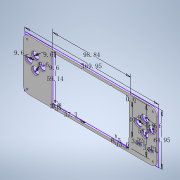
# Autodesk Inventor part: shell_panel
Saved by Autodesk Inventor 2022 (Build 260153000, 153)
## iProperties
Created: 2022-07-04
Part Number: shell_panel
Material: 常规
Document SubType Name: Modeling
Designer: yangmc
Density: 1 g/cm^3
Appearance: 默认
Author: yangmc
Autodesk Inventor part; units mm, degrees
ref_plane "YZ Plane" through (0, 0, 0) normal (1, 0, 0) x (0, 1, 0)
ref_plane "XZ Plane" through (0, 0, 0) normal (0, 1, 0) x (-1, 0, 0)
ref_plane "XY Plane" through (0, 0, 0) normal (0, 0, 1) x (1, 0, 0)
sketch "草图1" plane through (0, 0, 0) normal (0, 0, 1) x (1, 0, 0)
  circle A0 centre (15.38, 47) radius 4.8
  circle A1 centre (7.13, 38.85) radius 4.8
  circle A2 centre (15.38, 30.6) radius 4.8
  circle A3 centre (23.63, 38.85) radius 4.8
  circle A4 centre (154.65, 47) radius 4.8
  circle A5 centre (154.65, 30.5) radius 4.8
  circle A6 centre (162.9, 38.75) radius 4.8
  circle A7 centre (146.4, 38.75) radius 4.8
  line L0 (160.06, 15.83) -> (164.06, 15.83) construction
  line L1 (145.2, 15.83) -> (149.2, 15.83) construction
  line L2 (35.58, 3.33) -> (134.42, 3.33)
  line L3 (134.42, 3.33) -> (134.42, 61.67)
  line L4 (134.42, 61.67) -> (35.58, 61.67)
  line L5 (35.58, 61.67) -> (35.58, 3.33)
  line L6 (37.0724, 3.33) -> (39.6724, 3.33)
  line L7 (39.6724, 3.33) -> (39.6724, 2.53)
  line L8 (39.6724, 2.53) -> (37.0724, 2.53)
  line L9 (37.0724, 2.53) -> (37.0724, 3.33)
  line L10 (76.9724, 2.53) -> (74.3724, 2.53)
  line L11 (74.3724, 3.33) -> (76.9724, 3.33)
  line L12 (76.9724, 3.33) -> (76.9724, 2.53)
  line L13 (74.3724, 2.53) -> (74.3724, 3.33)
  line L14 (114.2724, 2.53) -> (111.6724, 2.53)
  line L15 (111.6724, 3.33) -> (114.2724, 3.33)
  line L16 (114.2724, 3.33) -> (114.2724, 2.53)
  line L17 (111.6724, 2.53) -> (111.6724, 3.33)
  line L18 (39.6724, 61.67) -> (37.0724, 61.67)
  line L19 (37.0724, 62.47) -> (39.6724, 62.47)
  line L20 (39.6724, 62.47) -> (39.6724, 61.67)
  line L21 (37.0724, 61.67) -> (37.0724, 62.47)
  line L22 (76.9724, 61.67) -> (74.3724, 61.67)
  line L23 (74.3724, 62.47) -> (76.9724, 62.47)
  line L24 (76.9724, 62.47) -> (76.9724, 61.67)
  line L25 (74.3724, 61.67) -> (74.3724, 62.47)
  line L26 (114.2724, 61.67) -> (111.6724, 61.67)
  line L27 (111.6724, 62.47) -> (114.2724, 62.47)
  line L28 (114.2724, 62.47) -> (114.2724, 61.67)
  line L29 (111.6724, 61.67) -> (111.6724, 62.47)
  line L30 (131.74, 3.33) -> (116.14, 3.33)
  line L31 (116.14, 3.33) -> (116.14, 2.83)
  line L32 (116.14, 2.83) -> (131.74, 2.83)
  line L33 (131.74, 2.83) -> (131.74, 3.33)
  line L34 (134.42, 16.2898) -> (135.02, 16.2898)
  line L35 (134.42, 43.8944) -> (134.42, 16.2898)
  line L36 (0.05, 0.05) -> (170, 0.05)
  line L37 (170, 0.05) -> (170, 65)
  line L38 (170, 65) -> (0.05, 65)
  line L39 (0.05, 65) -> (0.05, 0.05)
  line L40 (51, 0.05) -> (56.35, 0.05)
  line L41 (74.3724, 61.67) -> (76.72, 61.67)
  line L42 (143.65, 15.83) -> (150.75, 15.83) construction
  line L43 (145.2, 14.28) -> (149.2, 14.28)
  line L44 (149.2, 17.38) -> (145.2, 17.38)
  arc A8 (145.2, 17.38) -> (145.2, 14.28) centre (145.2, 15.83) ccw
  arc A9 (149.2, 14.28) -> (149.2, 17.38) centre (149.2, 15.83) ccw
  line L45 (158.51, 15.83) -> (165.61, 15.83) construction
  line L46 (160.06, 14.28) -> (164.06, 14.28)
  line L47 (164.06, 17.38) -> (160.06, 17.38)
  arc A10 (160.06, 17.38) -> (160.06, 14.28) centre (160.06, 15.83) ccw
  arc A11 (164.06, 14.28) -> (164.06, 17.38) centre (164.06, 15.83) ccw
  line L48 (135.02, 16.2898) -> (135.02, 56.2898)
  line L49 (135.02, 56.2898) -> (134.42, 56.2898)
  point P0 (0, 0)
  point P1 (162.06, 15.83)
  point P2 (147.2, 15.83)
  point P3 (72.9763, 65)
  point P4 (51, 0)
  point P5 (56.35, 0)
  point P6 (87, 65)
  point P7 (73, 65)
  point P8 (0, 0)
  point P9 (1.44, 58.34)
  point P10 (3.94, 58.34)
  point P11 (38.84, 58.34)
  point P12 (41.34, 58.34)
  point P13 (76.24, 58.34)
  point P14 (78.74, 58.34)
  point P15 (78.74, 0)
  point P16 (76.24, 0)
  point P17 (41.34, 0)
  point P18 (38.84, 0)
  point P19 (3.94, 0)
  point P20 (1.44, 0)
  point P21 (96.16, 0)
  point P22 (80.56, 0)
  point P23 (98.84, 43.1523)
  point P24 (37.02, 61.67)
  point P25 (39.52, 61.67)
  point P26 (74.42, 61.67)
  point P27 (76.92, 61.67)
  point P28 (111.82, 61.67)
  point P29 (114.32, 61.67)
  point P30 (114.32, 3.33)
  point P31 (111.82, 3.33)
  point P32 (76.92, 3.33)
  point P33 (74.42, 3.33)
  point P34 (39.52, 3.33)
  point P35 (37.02, 3.33)
  point P36 (39.6724, 3.33)
  point P37 (37.0724, 3.33)
  point P38 (76.9724, 3.33)
  point P39 (74.3724, 3.33)
  point P40 (114.2724, 3.33)
  point P41 (111.6724, 3.33)
  point P42 (111.6724, 61.67)
  point P43 (114.2724, 61.67)
  point P44 (74.3724, 61.67)
  point P45 (76.9724, 61.67)
  point P46 (37.0724, 61.67)
  point P47 (39.6724, 61.67)
  point P48 (147.2, 15.83)
  point P49 (162.06, 15.83)
  dimension "d2" = 9.6
  dimension "d3" = 9.6
  dimension "d4" = 9.6
  dimension "d5" = 9.6
  dimension "d6" = 9.6
  dimension "d7" = 9.6
  dimension "d8" = 9.6
  dimension "d9" = 9.6
  dimension "d10" = 2
  dimension "d12" = 2
  dimension "d22" = 98.84
  dimension "d23" = 58.34
  dimension "d24" = 2.6
  dimension "d25" = 0.8
  dimension "d26" = 37.3
  dimension "d27" = 59.14
  dimension "d28" = 15.6
  dimension "d29" = 0.5
  dimension "d31" = 169.95
  dimension "d32" = 64.95
  dimension "d43" = 7.1
  dimension "d44" = 3.1
  dimension "d45" = 7.1
  dimension "d46" = 3.1
  dimension "d64" = 40
  dimension "d65" = 0.6
  constraints: 108 end point, 12 centre point, 12 point on circle, 11 horizontal, 10 parallel, 10 point on line, 8 tangent, 5 perpendicular, 4 midpoint, 2 collinear, 1 vertical, 38 other
  measures "d2" diameter of A0
  measures "d3" diameter of A1
  measures "d4" diameter of A2
  measures "d5" diameter of A3
  measures "d6" diameter of A4
  measures "d7" diameter of A5
  measures "d8" diameter of A6
  measures "d9" diameter of A7
  measures "d10" distance of point (162.06, 15.83) L0.end
  measures "d12" distance of point (147.2, 15.83) L1.end
  measures "d22" distance of L4.end L3.end
  measures "d23" distance of L3.end L2.end
  measures "d24" distance of L7.end L8.end
  measures "d25" distance of L6.end L7.end
  measures "d26" distance of L7.end L10.start
  measures "d27" distance of L7.end L18.start
  measures "d28" distance of L32.end L31.end
  measures "d29" distance of L31.end L30.end
  measures "d31" distance of L38.end L37.end
  measures "d32" distance of L37.end L36.end
  measures "d43" distance of L42.start L42.end
  measures "d44" diameter of A9
  measures "d45" distance of L45.start L45.end
  measures "d46" diameter of A11
  measures "d64" distance of L34.end L48.end
  measures "d65" distance of L48.end L49.end
extrude "拉伸3" add sketch "草图1" along normal blind 2.2
extrude "拉伸4" add sketch "草图1" along normal blind 0.8 separate body contours L2 L7 L8 L9 | L21 L19 L20 L4 | L2 L12 L10 L13 | L25 L23 L24 L4 | L2 L16 L14 L17 | L29 L27 L28 L4
fillet "圆角1" radius 8 4 edges at (0.05, 65, 1.1) (0.05, 0.05, 1.1) (170, 65, 1.1) (170, 0.05, 1.1) curvature continuous yes
sketch "草图2" plane through (0, 0, 2.2) normal (0, 0, 1) x (1, 0, 0)
  circle A0 centre (5, 5) radius 0.6
  circle A1 centre (5, 60) radius 0.6
  circle A2 centre (165, 5) radius 0.6
  circle A3 centre (165, 60) radius 0.6
  point P0 (0, 0)
  point P1 (0, 0)
  dimension "d48" = 1.2
  dimension "d49" = 1.2
  dimension "d50" = 1.2
  dimension "d51" = 1.2
  constraints: 6 coincident, 4 centre point
  measures "d48" diameter of A0
  measures "d49" diameter of A1
  measures "d50" diameter of A2
  measures "d51" diameter of A3
hole "孔1" at (5, 60, 2.2) at (5, 5, 2.2) at (165, 5, 2.2) at (165, 60, 2.2) direction (0, 0, -1) diameter 1.2 end through all countersink diameter 2 countersink angle 90 bodies 1
sketch "草图3" plane through (0, 0, 0) normal (0, 0, 1) x (1, 0, 0)
  line L0 (0.05, 0.05) -> (34.55, 0.05)
  line L1 (34.55, 0.05) -> (34.55, 65)
  line L2 (34.55, 65) -> (0.05, 65)
  line L3 (0.05, 65) -> (0.05, 0.05)
  line L4 (136, 0.05) -> (170.0002, 0.05)
  line L5 (170.0002, 0.05) -> (170.0002, 65)
  line L6 (170.0002, 65) -> (136, 65)
  line L7 (136, 65) -> (136, 0.05)
  point P0 (0, 0)
  dimension "d59" = 34.5
  dimension "d60" = 64.95
  constraints: 16 end point, 4 parallel, 2 horizontal, 2 perpendicular
  measures "d59" distance of L2.end L1.end
  measures "d60" distance of L1.end L0.end
extrude "拉伸5" cut sketch "草图3" along normal blind 0.7 bodies 1
